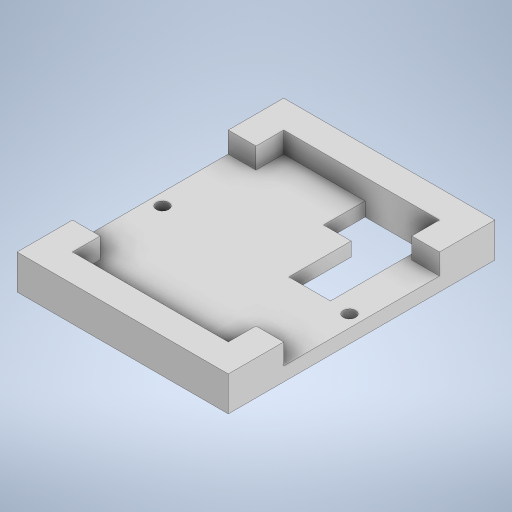
# Autodesk Inventor part: ESPLid
Saved by Autodesk Inventor 2023 (Build 270158000, 158)
## iProperties
Created: 2023-08-01
Part Number: ESPLid
Material: Generic
Document SubType Name: Modeling
Designer: campstudent
Density: 1 g/cm^3
Appearance: Default
Author: campstudent
Autodesk Inventor part; units mm, degrees
ref_plane "YZ Plane" through (0, 0, 0) normal (1, 0, 0) x (0, 1, 0)
ref_plane "XZ Plane" through (0, 0, 0) normal (0, 1, 0) x (-1, 0, 0)
ref_plane "XY Plane" through (0, 0, 0) normal (0, 0, 1) x (1, 0, 0)
sketch "Sketch1" plane through (0, 0, 0) normal (0, 1, 0) x (-1, 0, 0)
  line L0 (0, 0) -> (61, 0)
  line L1 (61, 0) -> (61, -77)
  line L2 (61, -77) -> (0, -77)
  line L3 (0, -77) -> (0, 0)
  line L4 (61, -35) -> (54, -35) construction
  line L5 (54, -35) -> (54, -42) construction
  line L6 (54, -42) -> (61, -42) construction
  line L7 (61, -42) -> (61, -35) construction
  line L8 (30.5, 0) -> (30.5, -77) construction
  line L9 (57.5, -35) -> (57.5, -42) construction
  line L10 (61, -38.5) -> (54, -38.5) construction
  circle A0 centre (57.5, -38.5) radius 1.8
  circle A1 centre (3.5, -38.5) radius 1.8
  dimension "d0" = 61
  dimension "d1" = 77
  dimension "d2" = 7
  dimension "d3" = 7
  dimension "d4" = 35
  dimension "d5" = 3.6
  constraints: 22 end point, 7 midpoint, 4 parallel, 2 centre point, 2 horizontal, 2 perpendicular, 1 point on line, 1 symmetric about line, 1 other
  measures "d0" distance between parallel lines of L3 L1
  measures "d1" distance of L0.end L1.end
  measures "d2" distance of L6.end L5.end
  measures "d3" distance of L5.end L4.end
  measures "d4" distance between parallel lines of L2 L6
  measures "d5" diameter of A0
extrude "Extrusion1" add sketch "Sketch1" along normal blind 4
sketch "Sketch2" plane through (0, 4, 0) normal (0, 1, 0) x (1, 0, 0)
  line L0 (-61, 77) -> (-61, 0) projected
  line L1 (-61, 0) -> (0, 0)
  line L2 (0, 0) -> (0, 8)
  line L3 (0, 8) -> (-61, 8)
  line L4 (-61, 8) -> (-61, 0)
  line L5 (-61, 0) -> (-53, 0)
  line L6 (-53, 0) -> (-53, 16)
  line L7 (-53, 16) -> (-61, 16)
  line L8 (-61, 16) -> (-61, 0)
  line L9 (-61, 0) -> (0, 0) projected
  line L10 (0, 0) -> (-8, 0)
  line L11 (-8, 0) -> (-8, 16)
  line L12 (-8, 16) -> (0, 16)
  line L13 (0, 16) -> (0, 0)
  line L14 (-61, 38.5) -> (0, 38.5) construction
  line L15 (0, 0) -> (0, 77) projected
  line L16 (-61, 77) -> (0, 77)
  line L17 (0, 77) -> (0, 69)
  line L18 (0, 69) -> (-61, 69)
  line L19 (-61, 69) -> (-61, 77)
  line L20 (-61, 77) -> (-53, 77)
  line L21 (-53, 77) -> (-53, 61)
  line L22 (-53, 61) -> (-61, 61)
  line L23 (-61, 61) -> (-61, 77)
  line L24 (-61, 77) -> (0, 77)
  line L25 (0, 77) -> (-8, 77)
  line L26 (-8, 77) -> (-8, 61)
  line L27 (-8, 61) -> (0, 61)
  line L28 (0, 61) -> (0, 77)
  point P0 (-8, 69)
  point P1 (0, 61)
  point P2 (-53, 69)
  point P3 (-8, 8)
  point P4 (-53, 8)
  dimension "d8" = 8
  dimension "d9" = 8
  dimension "d10" = 16
  dimension "d11" = 8
  dimension "d12" = 16
  constraints: 52 end point, 10 symmetric about line, 6 parallel, 3 horizontal, 3 perpendicular, 2 midpoint
  measures "d8" distance between parallel lines of L1 L3
  measures "d9" distance of L7.end L6.end
  measures "d10" distance of L6.end L5.end
  measures "d11" distance of L11.end L12.end
  measures "d12" distance of L10.end L11.end
extrude "Extrusion2" add sketch "Sketch2" along normal blind 6 contours L16 L21 L18 L0 | L18 L21 L22 L0 | L16 L26 L18 L21 | L16 L15 L18 L26 | L7 L6 L3 L0 | L18 L15 L27 L26 | L3 L6 L1 L0 | L3 L11 L1 L6 | L11 L12 L13 L3 | L3 L2 L1 L11
sketch "Sketch3" plane through (0, 4, 0) normal (0, 1, 0) x (1, 0, 0)
  line L0 (-51.5, 8) -> (-9.5, 8) construction
  line L1 (-9.5, 8) -> (-9.5, 69) construction
  line L2 (-9.5, 69) -> (-51.5, 69) construction
  line L3 (-51.5, 69) -> (-51.5, 8) construction
  line L4 (-61, 61) -> (-61, 16) projected
  line L5 (-61, 0) -> (0, 0) projected
  line L6 (-9.5, 69) -> (-21.5, 69)
  line L7 (-21.5, 69) -> (-21.5, 39)
  line L8 (-21.5, 39) -> (-9.5, 39)
  line L9 (-9.5, 39) -> (-9.5, 69)
  line L10 (-9.5, 66) -> (-9.5, 54)
  line L11 (-9.5, 69) -> (-29.5, 69)
  line L12 (-29.5, 69) -> (-29.5, 57)
  line L13 (-29.5, 57) -> (-9.5, 57)
  line L14 (-9.5, 57) -> (-9.5, 69)
  point P0 (-21.5, 57)
  dimension "d15" = 42
  dimension "d16" = 61
  dimension "d17" = 9.5
  dimension "d18" = 8
  dimension "d19" = 12
  dimension "d20" = 30
  dimension "d25" = 20
  dimension "d26" = 12
  constraints: 26 end point, 6 parallel, 3 horizontal, 3 perpendicular, 1 midpoint
  measures "d15" distance of L2.end L1.end
  measures "d16" distance of L1.end L0.end
  measures "d17" distance between parallel lines of L4 L3
  measures "d18" distance between parallel lines of L5 L0
  measures "d19" distance of L8.end L7.end
  measures "d20" distance of L7.end L6.end
  measures "d25" distance of L13.end L12.end
  measures "d26" distance of L12.end L11.end
extrude "Extrusion3" cut sketch "Sketch3" against normal through all
body "Solid1"
